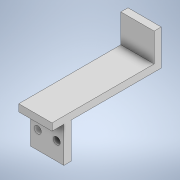
# Autodesk Inventor part: holder
Saved by Autodesk Inventor 2021 (Build 250183000, 183)
## iProperties
Created: 2021-01-07
Part Number: holder
Material: Generic
Document SubType Name: Modeling
Designer: awitc
Density: 1 g/cm^3
Appearance: Default
Author: awitc
Autodesk Inventor part; units mm, degrees
ref_plane "YZ Plane" through (0, 0, 0) normal (1, 0, 0) x (0, 1, 0)
ref_plane "XZ Plane" through (0, 0, 0) normal (0, 1, 0) x (-1, 0, 0)
ref_plane "XY Plane" through (0, 0, 0) normal (0, 0, 1) x (1, 0, 0)
sketch "Sketch1" plane through (0, 0, 0) normal (0, 1, 0) x (-1, 0, 0)
  line L0 (0, 0) -> (14, 0)
  line L1 (14, 0) -> (14, -35)
  line L2 (14, -35) -> (0, -35)
  line L3 (0, -35) -> (0, 0)
  line L4 (14, -35) -> (0, -35)
  line L5 (0, -35) -> (0, -38)
  line L6 (0, -38) -> (14, -38)
  line L7 (14, -38) -> (14, -35)
  line L8 (14, 0) -> (0, 0)
  line L9 (0, 0) -> (0, 3)
  line L10 (0, 3) -> (14, 3)
  line L11 (14, 3) -> (14, 0)
  dimension "d0" = 14
  dimension "d1" = 35
  dimension "d2" = 3
  dimension "d3" = 3
  constraints: 24 end point, 6 parallel, 3 horizontal, 3 perpendicular
  measures "d0" distance of L1.end L2.end
  measures "d1" distance of L0.end L1.end
  measures "d2" distance of L5.end L4.end
  measures "d3" distance of L8.end L9.end
extrude "Extrusion1" add sketch "Sketch1" along normal blind 3 contours L0 L1 L2 L3
extrude "Extrusion2" add sketch "Sketch1" along normal blind 15 contours L2 L7 L6 L5
extrude "Extrusion3" add sketch "Sketch1" along normal blind 3 and the other way blind 15 contours L9 L10 L11 L0
sketch "Sketch2" plane through (-14, 3, 3) normal (0, 0, 1) x (1, 0, 0)
  line L0 (0, 0) -> (14, 0) projected
  line L1 (14, 0) -> (14, -3)
  line L2 (14, -3) -> (0, -3)
  line L3 (0, -3) -> (0, 0)
  line L4 (0, 0) -> (14, 0)
  constraints: 8 end point, 2 parallel, 1 perpendicular, 1 vertical
extrude "Extrusion4" add sketch "Sketch2" along normal blind 5
sketch "Sketch3" plane through (-14, -15, 3) normal (0, 0, 1) x (1, 0, 0)
  line L0 (14, 0) -> (14, 15) projected
  line L1 (14, 15) -> (14, 11)
  line L2 (14, 0) -> (0, 0) projected
  line L3 (14, 0) -> (14, 4)
  line L4 (0, 0) -> (0, 15) projected
  line L5 (0, 0) -> (0, 4)
  line L6 (0, 15) -> (0, 11)
  line L7 (14, 7.5) -> (10, 7.5)
  line L8 (0, 7.5) -> (4, 7.5)
  line L9 (10, 7.5) -> (11, 7.5)
  circle A0 centre (11, 7.5) radius 1.5
  line L10 (4, 7.5) -> (1, 7.5)
  line L11 (4, 7.5) -> (3, 7.5)
  circle A1 centre (3, 7.5) radius 1.5
  dimension "d18" = 4
  dimension "d20" = 4
  dimension "d28" = 4
  dimension "d29" = 4
  dimension "d32" = 1
  dimension "d33" = 3
  dimension "d34" = 3
  dimension "d35" = 1
  dimension "d36" = 3
  constraints: 18 end point, 7 point on line, 4 coincident, 2 centre point, 2 horizontal, 2 midpoint
  measures "d18" distance of L2.end L5.end
  measures "d20" distance of L4.end L6.end
  measures "d28" distance of L7.start L7.end
  measures "d29" distance of L8.start L8.end
  measures "d32" distance of L9.start L9.end
  measures "d33" diameter of A0
  measures "d34" distance of L10.start L10.end
  measures "d35" distance of L10.start L11.end
  measures "d36" diameter of A1
extrude "Extrusion5" cut sketch "Sketch3" against normal blind 5
body "Solid1"
